Autodesk Fusion 360 part; units mm, degrees
note: some values were not read from the file. Set by a fixed rule: which face or edge a step refers to.
(part 2 of 2)
sketch "Sketch1 (3)" plane through (-90, 0, 0) normal (-1, 0, 0) x (0, -1, 0) in component "Connectors Mount"
  line L0 (67.5, -5.0963) -> (65.4615, 0)
  line L1 (65.4615, 0) -> (-61, 0)
  line L2 (-61, 0) -> (-61, -7.8)
  line L3 (-61, -7.8) -> (4, -7.8)
  line L4 (4, -7.8) -> (4, -5.8)
  line L5 (4, -5.8) -> (8.5, -5.8)
  line L6 (54, -5.8) -> (54, -7.8)
  line L7 (54, -7.8) -> (65, -7.8)
  line L8 (65, -7.8) -> (65, -15)
  line L9 (65, -15) -> (67.5, -15)
  line L10 (67.5, -15) -> (67.5, -5.0963)
  circle A0 centre (30, -3) radius 1.425
  circle A1 centre (-30, -3) radius 1.425
  line L11 (4, -7.8) -> (4, -15)
  line L12 (4, -7.8) -> (4, 0)
  line L13 (54, -7.8) -> (54, -15)
  line L14 (54, -15) -> (4, -15)
  line L15 (54, -7.8) -> (54, 0)
  circle A2 centre (30, -3) radius 1.65
  arc A3 (8.5, -5.8) -> (9, -5.3) centre (8.5, -5.3) ccw
  arc A4 (9.5, -4.8) -> (9, -5.3) centre (9.5, -5.3) ccw
  line L16 (9.5, -4.8) -> (18.5, -4.8)
  arc A5 (19, -5.3) -> (18.5, -4.8) centre (18.5, -5.3) ccw
  arc A6 (19, -5.3) -> (19.5, -5.8) centre (19.5, -5.3) ccw
  line L17 (19.5, -5.8) -> (54, -5.8)
  line L18 (4, -11.5) -> (54, -11.5)
  dimension "d86" = 3.3
  dimension "d183" = 11.5
  constraint coincident L3.end L4.start
  constraint perpendicular L3 L11
  constraint coincident L1 L12.end
  constraint perpendicular L1 L12
  constraint coincident L6.end L7.start
  constraint perpendicular L7 L13
  constraint perpendicular L6 L14
  constraint collinear L9 L14
  constraint coincident L1 L15.end
  constraint perpendicular L1 L15
  constraint concentric A0 A2
  constraint coincident L11 L18.start
  constraint coincident L13 L18.end
  constraint perpendicular L13 L18
  measures "d86" diameter of A2
  measures "d183" distance of L1 L18
extrude "Extrude1''" add sketch "Sketch1 (3)" along normal up to surface (18.55 mm away) separate body contours L1 L5 L12 L15 A3 A4 L16 A5 A6 L17 | L4 L5 L6 L11 L12 L13 L15 A3 A4 L16 A5 A6 L17 L18 makes body 3 in component "Connectors Mount"
sketch "Sketch2 (2)" plane through (-90, 0, 0) normal (1, 0, 0) x (0, 1, 0) in component "Connectors Mount"
  line L0 (-4, -11.5) -> (-4, 0)
  line L1 (-4, 0) -> (-54, 0)
  line L2 (-44.5, -11.5) -> (-44.5, -7.2)
  line L3 (-44.5, -7.2) -> (-20.2, -7.2)
  line L4 (-19.3, -5.5) -> (-9, -5.5)
  line L5 (-9, -5.5) -> (-9, -15)
  line L6 (-20.2, -7.2) -> (-20.2, -11.5)
  line L7 (-19.3, -5.5) -> (-19.3, -11.5)
  line L8 (-54, 0) -> (-54, -11.5)
  line L9 (-54, -11.5) -> (-4, -11.5)
  circle A0 centre (-30, -3) radius 1.65
  dimension "d89" = 7.2
  dimension "d92" = 5.5
  dimension "d106" = 24.3
  dimension "d107" = 35.5
  dimension "d108" = 10.3
  dimension "d184" = 9.5
  constraint perpendicular L2 L3
  constraint coincident L2.start L9
  constraint coincident L6.end L9
  constraint perpendicular L6 L9
  constraint coincident L7.end L9
  constraint perpendicular L7 L9
  measures "d89" distance of L1 L3
  measures "d92" distance of L1 L4
  measures "d106" distance of L2.end L3.end
  measures "d107" distance of L2 L5
  measures "d108" distance of L4.start L4.end
  measures "d184" distance of L2 L8
extrude "Extrude2'" cut sketch "Sketch2 (2)" against normal up to surface (18.55 mm away) contours L4 L5 L7 L9 | L2 L3 L6 L9 bodies 3 in component "Connectors Mount"
sketch "Sketch3 (3)" plane through (-108.55, 0, 0) normal (-1, 0, 0) x (0, -1, 0) in component "Connectors Mount"
  line L0 (9, -11.5) -> (9, -5.5)
  line L1 (9, -5.5) -> (19.3, -5.5)
  line L2 (19.3, -5.5) -> (19.3, -11.5)
  line L3 (20.2, -11.5) -> (20.2, -7.2)
  line L4 (20.2, -7.2) -> (44.5, -7.2)
  line L5 (44.5, -7.2) -> (44.5, -11.5)
  line L6 (54, 0) -> (4, 0)
  line L7 (4, 0) -> (4, -11.5)
  line L8 (19.3, -11.5) -> (20.2, -11.5)
  line L9 (44.5, -11.5) -> (54, -11.5)
  line L10 (54, -11.5) -> (54, 0)
  line L11 (4, -11.5) -> (9, -11.5)
  line L12 (21.7, -11.5) -> (20.2, -11.5)
  arc A0 (23.2, -8.5) -> (21.7, -10) centre (23.2, -10) ccw
  line L13 (21.7, -10) -> (21.7, -11.5)
  circle A1 centre (30, -3) radius 1.65
  line L14 (23.2, -8.5) -> (26.2, -8.5)
  line L15 (26.2, -8.5) -> (26.2, -7.2)
  dimension "d186" = 1.5
  dimension "d188" = 3
  dimension "d217" = 1.5
  dimension "d218" = 6
  constraint coincident L3.start L8.end
  constraint perpendicular L3 L12
  constraint tangent A0 L13
  constraint perpendicular L12 L13
  constraint tangent A0 L14
  constraint coincident L4 L15.end
  constraint perpendicular L4 L15
  constraint horizontal L14
  measures "d186" radius of A0
  measures "d188" distance of L3 A0.centre
  measures "d217" distance of L12 A0.centre
  measures "d218" distance of L3 L15
extrude "Extrude3''" add sketch "Sketch3 (3)" against normal blind 1.5 contours L3 L4 L12 A0 L13 L14 L15 bodies 3 in component "Connectors Mount"
sketch "Sketch4 (3)" plane through (-108.55, 0, 0) normal (-1, 0, 0) x (0, -1, 0) in component "Connectors Mount"
  line L0 (9, -11.5) -> (9, -5.5)
  line L1 (9, -5.5) -> (19.3, -5.5)
  line L2 (19.3, -5.5) -> (19.3, -11.5)
  line L3 (54, 0) -> (4, 0)
  line L4 (4, 0) -> (4, -11.5)
  circle A0 centre (14.15, -8.5) radius 3.5
  line L5 (14.15, -5.5) -> (14.15, -8.5) construction
  line L6 (17.65, -8.5) -> (17.65, -11.5201)
  line L7 (17.65, -11.5201) -> (19.3, -11.5)
  line L8 (10.65, -8.5) -> (10.65, -11.5)
  line L9 (10.65, -11.5) -> (9, -11.5)
  line L10 (19.3, -11.5) -> (21.7, -11.5)
  line L11 (54, -11.5) -> (54, 0)
  line L12 (21.7, -11.5) -> (21.7, -10)
  arc A1 (23.2, -8.5) -> (21.7, -10) centre (23.2, -10) ccw
  line L13 (23.2, -8.5) -> (26.2, -8.5)
  line L14 (26.2, -8.5) -> (26.2, -7.2)
  line L15 (26.2, -7.2) -> (44.5, -7.2)
  line L16 (44.5, -7.2) -> (44.5, -11.5)
  line L17 (44.5, -11.5) -> (54, -11.5)
  line L18 (4, -11.5) -> (9, -11.5)
  circle A2 centre (30, -3) radius 1.65
  dimension "d121" = 7
  dimension "d122" = 3
  constraint midpoint L1 L5.start
  constraint coincident A0.centre L5.end
  constraint perpendicular L1 L5
  constraint coincident A0 L6.start
  constraint perpendicular L1 L6
  constraint coincident L2.end L7.end
  constraint coincident A0 L8.start
  constraint coincident L0.start L9.end
  constraint perpendicular L0 L9
  constraint tangent A0 L8
  constraint tangent A0 L6
  measures "d121" diameter of A0
  measures "d122" distance of L5.start A0.centre
extrude "Extrude5''" cut sketch "Sketch4 (3)" against normal blind 15 contours L1 A0 picked at (14.4477, -5.2721) bodies 3 in component "Connectors Mount"
sketch "Sketch5 (3)" plane through (0, -20.2, 0) normal (0, -1, 0) x (1, 0, 0) in component "Connectors Mount"
  line L0 (-107.05, -11.5) -> (-90, -11.5)
  line L1 (-90, -11.5) -> (-90, -7.2)
  line L2 (-90, -7.2) -> (-107.05, -7.2)
  line L3 (-91, -7.2) -> (-91, -11.5)
  line L4 (-107.05, -7.2) -> (-107.05, -11.5)
  dimension "d192" = 1
  constraint coincident L2 L3.start
  constraint coincident L0 L3.end
  constraint perpendicular L0 L3
  measures "d192" distance of L1 L3
extrude "Extrude6''" add sketch "Sketch5 (3)" along normal blind 1 contours L0 L1 L2 L3 bodies 3 in component "Connectors Mount"
fillet "Fillet8'" radius 1 8 edges at (-99.275, -54, 0) (-99.275, -4, 0) (-90, -4, -5.75) (-90, -29, 0) (-90, -54, -5.75) (-108.55, -54, -5.75) (-108.55, -29, 0) (-108.55, -4, -5.75) on bodies 3 in component "Connectors Mount"
sketch "Sketch2 (3)" plane through (0, 0, -7.8) normal (0, 0, -1) x (1, 0, 0) in component "Bottom"
  circle A0 centre (60, 60) radius 1.65
  circle A1 centre (60, -60) radius 1.65
  circle A2 centre (-60, 60) radius 1.65
  circle A3 centre (-60, -60) radius 1.65
  arc A4 (-73.75, 56) -> (-71.75, 54) centre (-71.75, 56) ccw
  line L0 (-71.75, 54) -> (71.75, 54)
  arc A5 (71.75, 54) -> (73.75, 56) centre (71.75, 56) ccw
  line L1 (73.75, 56) -> (73.75, 61)
  arc A6 (75.75, 63) -> (73.75, 61) centre (75.75, 61) ccw
  line L2 (75.75, 63) -> (86, 63)
  arc A7 (88, 61) -> (86, 63) centre (86, 61) ccw
  line L3 (88, 61) -> (88, -61)
  arc A8 (86, -63) -> (88, -61) centre (86, -61) ccw
  line L4 (86, -63) -> (75.75, -63)
  arc A9 (73.75, -61) -> (75.75, -63) centre (75.75, -61) ccw
  line L5 (73.75, -61) -> (73.75, -56)
  arc A10 (73.75, -56) -> (71.75, -54) centre (71.75, -56) ccw
  line L6 (71.75, -54) -> (-71.75, -54)
  arc A11 (-71.75, -54) -> (-73.75, -56) centre (-71.75, -56) ccw
  line L7 (-73.75, -56) -> (-73.75, -61)
  arc A12 (-75.75, -63) -> (-73.75, -61) centre (-75.75, -61) ccw
  line L8 (-75.75, -63) -> (-86, -63)
  arc A13 (-88, -61) -> (-86, -63) centre (-86, -61) ccw
  line L9 (-88, -61) -> (-88, 4)
  line L10 (-88, 4) -> (-90, 4)
  line L11 (-90, 4) -> (-90, -61)
  arc A14 (-90, -61) -> (-86, -65) centre (-86, -61) ccw
  line L12 (-86, -65) -> (86, -65)
  arc A15 (86, -65) -> (90, -61) centre (86, -61) ccw
  line L13 (90, -61) -> (90, 65)
  line L14 (90, 65) -> (-90, 65)
  line L15 (-90, 65) -> (-90, 54)
  line L16 (-90, 54) -> (-88, 54)
  line L17 (-88, 54) -> (-88, 61)
  arc A16 (-86, 63) -> (-88, 61) centre (-86, 61) ccw
  line L18 (-86, 63) -> (-75.75, 63)
  arc A17 (-73.75, 61) -> (-75.75, 63) centre (-75.75, 61) ccw
  line L19 (-73.75, 61) -> (-73.75, 56)
  circle A18 centre (78.5, 57.5) radius 1.65 construction
  circle A19 centre (78.5, 57.5) radius 1.65 construction
  circle A20 centre (-78.5, 57.5) radius 1.65 construction
  circle A21 centre (-78.5, 57.5) radius 1.65 construction
  circle A22 centre (-78.5, -57.5) radius 1.65 construction
  circle A23 centre (-78.5, -57.5) radius 1.65 construction
  circle A24 centre (78.5, -57.5) radius 1.65 construction
  circle A25 centre (78.5, -57.5) radius 1.65 construction
  circle A26 centre (-78.5, 57.5) radius 3.25
  circle A27 centre (78.5, 57.5) radius 3.25
  circle A28 centre (78.5, -57.5) radius 3.25
  circle A29 centre (-78.5, -57.5) radius 3.25
  line L20 (-81.75, 6) -> (-81.75, -51.2752)
  line L21 (-81.75, -51.2752) -> (81.75, -51.2752)
  line L22 (81.75, -51.2752) -> (81.75, 52)
  line L23 (81.75, 52) -> (-90, 52)
  line L24 (-90, 52) -> (-90, 54)
  line L25 (83.75, 53) -> (83.75, -53) construction
  line L26 (-83.75, -53) -> (-83.75, 8.5) construction
  line L27 (-81.75, 6) -> (-90, 6)
  line L28 (-90, 6) -> (-90, 4)
  dimension "d133" = 6.5
  dimension "d134" = 2
  dimension "d135" = 2
  dimension "d136" = 2.7248
  dimension "d137" = 2
  dimension "d146" = 2
  constraint concentric A20 A26
  constraint concentric A18 A27
  constraint concentric A24 A28
  constraint concentric A22 A29
  constraint equal A28 A29
  constraint equal A27 A28
  constraint equal A26 A27
  constraint perpendicular L10 L20
  constraint perpendicular L9 L21
  constraint perpendicular L6 L22
  constraint perpendicular L9 L23
  constraint coincident L15.end L16.start
  constraint collinear L15 L24
  constraint perpendicular L20 L27
  constraint coincident L10.end L11.start
  constraint collinear L11 L28
  measures "d133" diameter of A26
  measures "d134" distance of L0 L23
  measures "d135" distance of L22 L25
  measures "d136" distance of L6 L21
  measures "d137" distance of L20 L26
  measures "d146" distance of L27.end L10.end
extrude "Extrude2''" add sketch "Sketch2 (3)" along normal blind 9.5 separate body makes body 4 in component "Bottom"
sketch "Sketch3 (4)" plane through (0, 0, -17.3) normal (0, 0, -1) x (1, 0, 0) in component "Bottom"
  circle A0 centre (-60, -60) radius 1.65
  circle A1 centre (60, 60) radius 1.65
  circle A2 centre (60, -60) radius 1.65
  circle A3 centre (78.5, -57.5) radius 3.25
  circle A4 centre (-78.5, -57.5) radius 3.25
  circle A5 centre (-78.5, 57.5) radius 3.25
  circle A6 centre (78.5, 57.5) radius 3.25
  circle A7 centre (-60, 60) radius 1.65
  line L0 (-90, 4) -> (-90, -61)
  arc A8 (-90, -61) -> (-86, -65) centre (-86, -61) ccw
  line L1 (-86, -65) -> (86, -65)
  arc A9 (86, -65) -> (90, -61) centre (86, -61) ccw
  line L2 (90, -61) -> (90, 65)
  line L3 (90, 65) -> (-90, 65)
  line L4 (-90, 65) -> (-90, 54)
  line L5 (-90, 54) -> (-90, 52)
  line L6 (-90, 52) -> (81.75, 52)
  line L7 (81.75, 52) -> (81.75, -51.2752)
  line L8 (81.75, -51.2752) -> (-81.75, -51.2752)
  line L9 (-81.75, -51.2752) -> (-81.75, 6)
  line L10 (-90, 4) -> (-90, 52)
  line L11 (-81.75, 6) -> (-90, 6)
  line L12 (-90, 6) -> (-90, 4)
  constraint coincident L0.start L10.start
  constraint coincident L5.end L6.start
extrude "Extrude3'''" add sketch "Sketch3 (4)" along normal blind 3 contours A3 | A4 | A5 | A6 | L0 A8 L1 A9 L2 L3 L4 L5 L6 L7 L8 L9 L10 L11 L12 | L6 L7 L8 L9 L10 L11 bodies 4 in component "Bottom"
sketch "Sketch4 (4)" plane through (0, 0, -20.3) normal (0, 0, -1) x (1, 0, 0) in component "Bottom"
  circle A0 centre (60, 60) radius 1.65
  circle A1 centre (-60, 60) radius 1.65
  circle A2 centre (-60, -60) radius 1.65
  circle A3 centre (60, -60) radius 1.65
  arc A4 (-90, -61) -> (-86, -65) centre (-86, -61) ccw
  line L0 (-86, -65) -> (86, -65)
  arc A5 (86, -65) -> (90, -61) centre (86, -61) ccw
  line L1 (90, -61) -> (90, 65)
  line L2 (90, 65) -> (-90, 65)
  line L3 (-90, 65) -> (-90, 54)
  line L4 (-90, 54) -> (-90, 52)
  line L5 (-90, 4) -> (-90, -61)
  line L6 (-108.75, 31.65) -> (-108.75, 28.35) construction
  line L7 (-108.75, 54) -> (-108.75, 4) construction
  line L8 (-108.75, 4) -> (-108.75, 54) construction
  line L9 (-108.75, 54) -> (-108.75, 4)
  line L10 (-108.75, 4) -> (-90, 4)
  line L11 (-90.6, 4) -> (-108.75, 4) construction
  circle A6 centre (-99.375, 49) radius 1.65
  circle A7 centre (-99.375, 9) radius 1.65
  line L12 (-108.75, 29) -> (-95, 29) construction
  line L13 (-99.375, 4) -> (-99.375, 29.3924) construction
  line L14 (-90, 6) -> (-90, 4)
  line L15 (-108.75, 54) -> (-90, 54)
  line L16 (-90, 52) -> (-90, 6)
  dimension "d142" = 40
  dimension "d143" = 3.3
  constraint perpendicular L2 L9
  constraint collinear L10 L11
  constraint collinear L8 L9
  constraint midpoint L9 L12.start
  constraint perpendicular L7 L12
  constraint midpoint L10 L13.start
  constraint coincident A7.centre L13
  constraint symmetric A6 A7 L12
  constraint coincident L7.start L8.end
  constraint coincident L3.end L4.start
  constraint vertical L13
  constraint coincident L5.start L10.end
  measures "d142" distance of A6.centre A7.centre
  measures "d143" diameter of A7
extrude "Extrude4''" add sketch "Sketch4 (4)" against normal up to surface (3 mm away) contours L4 L9 L10 L14 L15 L16 bodies 4 in component "Bottom"
fillet "Fillet1'" radius 4 1 edges at (90, -65, -14.05) on bodies 4 in component "Bottom"
sketch "Sketch5 (4)" plane through (0, 0, -17.3) normal (0, 0, 1) x (-1, 0, 0) in component "Bottom"
  line L0 (108.75, 4) -> (108.75, 54)
  line L1 (90, 54) -> (90, 52)
  line L2 (90, 52) -> (-81.75, 52)
  line L3 (-81.75, 52) -> (-81.75, -51.2752)
  line L4 (-81.75, -51.2752) -> (81.75, -51.2752)
  line L5 (81.75, -51.2752) -> (81.75, 6)
  line L6 (81.75, 6) -> (90, 6)
  line L7 (90, 6) -> (90, 4)
  line L8 (90, 4) -> (108.75, 4)
  circle A0 centre (99.375, 49) radius 1.65
  circle A1 centre (99.375, 9) radius 1.65
  circle A2 centre (19, -24.5) radius 1.375
  circle A3 centre (-39, -24.5) radius 1.375
  circle A4 centre (-39, 24.5) radius 1.375
  circle A5 centre (19, 24.5) radius 1.375
  circle A6 centre (19, 24.5) radius 2.5
  circle A7 centre (-39, 24.5) radius 2.5
  circle A8 centre (-39, -24.5) radius 2.5
  circle A9 centre (19, -24.5) radius 2.5
  line L9 (108.75, 54) -> (90, 54)
  dimension "d151" = 19
  dimension "d152" = 39
  dimension "d154" = 24.5
  dimension "d155" = 24.5
  dimension "d156" = 2.75
  dimension "d170" = 5
  constraint horizontal A2.centre A3.centre
  constraint equal A4 A5
  constraint equal A3 A4
  constraint equal A2 A3
  constraint vertical A2.centre A5.centre
  constraint vertical A3.centre A4.centre
  constraint horizontal A4.centre A5.centre
  constraint concentric A5 A6
  constraint concentric A4 A7
  constraint concentric A3 A8
  constraint concentric A2 A9
  constraint equal A8 A9
  constraint equal A7 A8
  constraint equal A6 A7
  measures "d151" horizontal distance of origin A2.centre
  measures "d152" horizontal distance of origin A3.centre
  measures "d154" vertical distance of origin A3.centre
  measures "d155" vertical distance of origin A4.centre
  measures "d156" diameter of A5
  measures "d170" diameter of A6
extrude "Extrude5'''" cut sketch "Sketch5 (4)" against normal up to surface (3 mm away) contours A2 | A3 | A4 | A5 bodies 4 in component "Bottom"
extrude "Extrude8'" add sketch "Sketch5 (4)" along normal up to surface (3.5 mm away) contours A6 | A7 | A8 | A9 bodies 4 in component "Bottom"
sketch "Sketch8 (2)" plane through (0, 0, -20.3) normal (0, 0, -1) x (1, 0, 0) in component "Bottom"
  circle A0 centre (-19, 24.5) radius 1.375
  circle A1 centre (39, 24.5) radius 1.375
  circle A2 centre (-19, -24.5) radius 1.375
  circle A3 centre (39, -24.5) radius 1.375
  arc A4 (90, 61) -> (86, 65) centre (86, 61) ccw
  line L0 (86, 65) -> (-90, 65)
  line L1 (-90, 65) -> (-90, 54)
  line L2 (-90, 54) -> (-108.75, 54)
  line L3 (-108.75, 54) -> (-108.75, 4)
  line L4 (-108.75, 4) -> (-90, 4)
  line L5 (-90, 4) -> (-90, -61)
  arc A5 (-90, -61) -> (-86, -65) centre (-86, -61) ccw
  line L6 (-86, -65) -> (86, -65)
  arc A6 (86, -65) -> (90, -61) centre (86, -61) ccw
  line L7 (90, -61) -> (90, 61)
  circle A7 centre (-60, -60) radius 1.65
  circle A8 centre (60, 60) radius 1.65
  circle A9 centre (-60, 60) radius 1.65
  circle A10 centre (60, -60) radius 1.65
  circle A11 centre (-99.375, 49) radius 1.65
  circle A12 centre (-99.375, 9) radius 1.65
  circle A13 centre (39, 24.5) radius 2.5
  circle A14 centre (-19, 24.5) radius 2.5
  circle A15 centre (-19, -24.5) radius 2.5
  circle A16 centre (39, -24.5) radius 2.5
  dimension "d213" = 5
  constraint concentric A1 A13
  constraint concentric A0 A14
  constraint concentric A2 A15
  constraint concentric A3 A16
  constraint equal A13 A14
  constraint equal A14 A15
  constraint equal A15 A16
  measures "d213" diameter of A13
extrude "Extrude10'" cut sketch "Sketch8 (2)" against normal up to surface (2.5 mm away) contours A13 | A14 | A15 | A16 bodies 4 in component "Bottom"
sketch "Sketch6 (2)" plane through (0, 0, -17.3) normal (0, 0, 1) x (-1, 0, 0) in component "Bottom"
  line L0 (108.75, 4) -> (108.75, 54)
  line L1 (90, 54) -> (90, 52)
  line L2 (90, 52) -> (-81.75, 52)
  line L3 (-81.75, 52) -> (-81.75, -51.2752)
  line L4 (-81.75, -51.2752) -> (81.75, -51.2752)
  line L5 (81.75, -51.2752) -> (81.75, 6)
  line L6 (81.75, 6) -> (90, 6)
  line L7 (90, 6) -> (90, 4)
  line L8 (90, 4) -> (108.75, 4)
  circle A0 centre (99.375, 49) radius 1.65
  circle A1 centre (99.375, 9) radius 1.65
  line L9 (25, -20) -> (-25, -20) construction
  line L10 (-25, -20) -> (-25, 20) construction
  line L11 (-25, 20) -> (25, 20) construction
  line L12 (25, 20) -> (25, -20) construction
  line L13 (0, 0) -> (-48.8562, 0) construction
  circle A2 centre (-25, -20) radius 4
  circle A3 centre (-25, 20) radius 4
  line L14 (0, 0) -> (0, -41.4646) construction
  circle A4 centre (-19, -24.5) radius 2.75 construction
  circle A5 centre (25, -20) radius 4
  circle A6 centre (25, 20) radius 4
  circle A7 centre (-25, -20) radius 1.65
  circle A8 centre (-25, 20) radius 1.65
  circle A9 centre (25, 20) radius 1.65
  circle A10 centre (25, -20) radius 1.65
  line L15 (-26.5588, -17.3) -> (-28.1177, -20)
  line L16 (-28.1177, -20) -> (-26.5588, -22.7)
  line L17 (-26.5588, -22.7) -> (-23.4412, -22.7)
  line L18 (-23.4412, -22.7) -> (-21.8823, -20)
  line L19 (-21.8823, -20) -> (-23.4412, -17.3)
  line L20 (-23.4412, -17.3) -> (-26.5588, -17.3)
  line L21 (23.4412, -17.3) -> (21.8823, -20)
  line L22 (21.8823, -20) -> (23.4412, -22.7)
  line L23 (23.4412, -22.7) -> (26.5588, -22.7)
  line L24 (26.5588, -22.7) -> (28.1177, -20)
  line L25 (28.1177, -20) -> (26.5588, -17.3)
  line L26 (26.5588, -17.3) -> (23.4412, -17.3)
  line L27 (23.4412, 22.7) -> (21.8823, 20)
  line L28 (21.8823, 20) -> (23.4412, 17.3)
  line L29 (23.4412, 17.3) -> (26.5588, 17.3)
  line L30 (26.5588, 17.3) -> (28.1177, 20)
  line L31 (28.1177, 20) -> (26.5588, 22.7)
  line L32 (26.5588, 22.7) -> (23.4412, 22.7)
  line L33 (-26.5588, 22.7) -> (-28.1177, 20)
  line L34 (-28.1177, 20) -> (-26.5588, 17.3)
  line L35 (-26.5588, 17.3) -> (-23.4412, 17.3)
  line L36 (-23.4412, 17.3) -> (-21.8823, 20)
  line L37 (-21.8823, 20) -> (-23.4412, 22.7)
  line L38 (-23.4412, 22.7) -> (-26.5588, 22.7)
  circle A11 centre (-39, -24.5) radius 2.5
  circle A12 centre (19, -24.5) radius 2.5
  circle A13 centre (-39, 24.5) radius 2.5
  circle A14 centre (19, 24.5) radius 2.5
  line L39 (108.75, 54) -> (90, 54)
  point P0 (-25, -20)
  point P1 (25, -20)
  point P2 (25, 20)
  point P3 (-25, 20)
  dimension "d159" = 50
  dimension "d160" = 8
  dimension "d162" = 40
  dimension "d163" = 5.5
  dimension "d164" = 3.3
  dimension "d167" = 2.7
  constraint horizontal L9
  constraint vertical L10
  constraint horizontal L11
  constraint vertical L12
  constraint coincident L13.start L14.start
  constraint horizontal L13
  constraint symmetric L9 L11 L13
  constraint coincident P0 L9.end
  constraint coincident P3 L10.end
  constraint perpendicular L13 L14
  constraint symmetric L10 L12 L14
  constraint coincident P1 L9.start
  constraint coincident P2 L11.end
  constraint concentric A2 A7
  constraint equal A2 A3
  constraint equal A3 A6
  constraint equal A5 A6
  constraint concentric A3 A8
  constraint concentric A6 A9
  constraint concentric A5 A10
  constraint equal A7 A10
  constraint equal A9 A10
  constraint equal A8 A9
  constraint horizontal L20
  constraint equal L32 L38
  constraint equal L26 L32
  constraint equal L20 L26
  constraint horizontal L26
  constraint horizontal L32
  constraint horizontal L38
  measures "d159" distance of P1 P0
  measures "d160" diameter of A2
  measures "d162" distance of P0 P3
  measures "d163" diameter of A4
  measures "d164" diameter of A7
  measures "d167" distance of P0 L20
extrude "Extrude6'''" cut sketch "Sketch6 (2)" against normal up to surface (3 mm away) contours A7 | A8 | A9 | A10 bodies 4 in component "Bottom"
extrude "Extrude7'" add sketch "Sketch6 (2)" along normal blind 3 contours A2 | A3 | A5 | A6 bodies 4 in component "Bottom"
sketch "Sketch7 (2)" plane through (0, 0, -17.3) normal (0, 0, 1) x (-1, 0, 0) in component "Bottom"
  circle A0 centre (25, 20) radius 4
  circle A1 centre (-25, 20) radius 4
  circle A2 centre (-39, -24.5) radius 2.5
  circle A3 centre (19, -24.5) radius 2.5
  circle A4 centre (-39, 24.5) radius 2.5
  circle A5 centre (19, 24.5) radius 2.5
  line L0 (108.75, 4) -> (108.75, 54)
  line L1 (90, 54) -> (90, 52)
  line L2 (90, 52) -> (-81.75, 52)
  line L3 (-81.75, 52) -> (-81.75, -51.2752)
  line L4 (-81.75, -51.2752) -> (81.75, -51.2752)
  line L5 (81.75, -51.2752) -> (81.75, 6)
  line L6 (81.75, 6) -> (90, 6)
  line L7 (90, 6) -> (90, 4)
  line L8 (90, 4) -> (108.75, 4)
  circle A6 centre (99.375, 49) radius 1.65
  circle A7 centre (99.375, 9) radius 1.65
  circle A8 centre (-25, -20) radius 4
  circle A9 centre (25, -20) radius 4
  line L9 (-21, -51.2752) -> (-21, 52)
  line L10 (-29, 52) -> (-29, -51.2752)
  line L11 (29, -51.2752) -> (29, 52)
  line L12 (21, 52) -> (21, -51.2752)
  line L13 (108.75, 54) -> (90, 54)
  constraint coincident L4 L9.start
  constraint coincident L2 L9.end
  constraint coincident L2 L10.start
  constraint coincident L4 L10.end
  constraint perpendicular L4 L10
  constraint coincident L4 L11.start
  constraint coincident L2 L11.end
  constraint perpendicular L2 L11
  constraint coincident L2 L12.start
  constraint coincident L4 L12.end
  constraint perpendicular L4 L12
  constraint perpendicular L4 L9
  constraint tangent A8 L9
  constraint tangent A8 L10
  constraint tangent A9 L12
  constraint tangent A9 L11
extrude "Extrude9'" add sketch "Sketch7 (2)" along normal blind 2 contours A0 A9 L11 L12 | A0 A5 L2 L11 L12 | A3 L4 A9 L11 L12 | A5 L12 | A3 L12 | A1 L2 L9 L10 | L4 A8 L9 L10 | A1 A8 L9 L10 picked at (21.2565, 24.2879) picked at (21.2565, -24.7121) bodies 4 in component "Bottom"
fillet "Fillet3'" radius 2 4 edges at (-81.75, 51.2752, -12.55) (-81.75, -6, -12.55) (81.75, 51.2752, -12.55) (81.75, -52, -12.55) on bodies 4 in component "Bottom"
fillet "Fillet4'" radius 1 9 edges at (-29, -0.3624, -17.3) (-59.5, -52, -17.3) (-54.375, 51.2752, -17.3) (-81.1642, 50.6894, -17.3) (-81.75, 22.6376, -17.3) (-82.3358, -5.4142, -17.3) (-86.875, -6, -17.3) (-16.6692, 23.596, -17.3) (-16.6692, -25.404, -17.3) 2 faces at (8.4203, -8.0527, -17.3) (68.2508, -8.0467, -17.3) on bodies 4 in component "Bottom"
fillet "Fillet5" radius 1 8 edges at (25, 16, -15.3) (25, -24, -15.3) (-25, -24, -15.3) (-25, 16, -15.3) (25, 24, -15.3) (-25, 24, -15.3) (-25, -16, -15.3) (25, -16, -15.3) on bodies 4 in component "Bottom"
sketch "Sketch1 (4)" plane through (-108.75, 0, 0) normal (-1, 0, 0) x (0, -1, 0) in component "Connectors Mount Bottom"
  line L0 (54, -17.3) -> (4, -17.3)
  line L1 (4, -17.3) -> (4, -20.3)
  line L2 (4, -20.3) -> (54, -20.3)
  line L3 (54, -20.3) -> (54, -17.3)
  arc A0 (15.9528, -5.5) -> (12.3472, -5.5) centre (14.15, -8.5) ccw
  arc A1 (23.2, -8.5) -> (21.7, -10) centre (23.2, -10) ccw
  line L4 (21.7, -10) -> (21.7, -11.5)
  line L5 (54, -17.3) -> (54, -11.5)
  circle A2 centre (14.15, -8.5) radius 3.5
  line L6 (21.7, -11.5) -> (15.9528, -11.5)
  line L7 (12.3472, -11.5) -> (4, -11.5)
  line L8 (4, -11.5) -> (4, -17.3)
  line L9 (23.2, -8.5) -> (26.2, -8.5)
  line L10 (26.2, -8.5) -> (26.2, -7.2)
  line L11 (26.2, -7.2) -> (44.5, -7.2)
  line L12 (44.5, -7.2) -> (44.5, -11.5)
  line L13 (21.7, -13) -> (21.7, -11.5)
  arc A3 (21.7, -13) -> (23.2, -14.5) centre (23.2, -13) ccw
  line L14 (23.2, -14.5) -> (26.2, -14.5)
  line L15 (26.2, -14.5) -> (26.2, -15.8)
  line L16 (26.2, -15.8) -> (44.5, -15.8)
  line L17 (44.5, -15.8) -> (44.5, -11.5)
  line L18 (44.5, -11.5) -> (54, -11.5)
  constraint coincident L0.start L3.end
  constraint perpendicular L0 L5
  constraint concentric A0 A2
  constraint equal A0 A2
  constraint coincident L4.end L6.start
  constraint coincident A2 L6.end
  constraint perpendicular L4 L6
  constraint coincident A2 L7.start
  constraint horizontal L7
  constraint coincident L0.end L1.start
  constraint collinear L6 L7
  constraint perpendicular L7 L8
  constraint symmetric A1.start L6 A3.end
  constraint symmetric A1.end L6 L13.start
  constraint symmetric A1 L6 A3
  constraint symmetric L4.end L6 L13.end
  constraint symmetric L6 A1.start A3.end
  constraint symmetric L6 L9.end L14.end
  constraint symmetric L6 L10.end L15.end
  constraint symmetric L6 L11.end L16.end
  constraint symmetric L6 L12.end L17.end
  constraint coincident L12.end L17.end
  constraint perpendicular L5 L18
extrude "Extrude1'''" add sketch "Sketch1 (4)" against normal up to surface (18.75 mm away) separate body contours L0 L5 A2 L6 L7 L8 L13 A3 L14 L15 L16 L17 L18 makes body 5 in component "Connectors Mount Bottom"
sketch "Sketch2 (4)" plane through (0, 0, -17.3) normal (0, 0, -1) x (1, 0, 0) in component "Connectors Mount Bottom"
  line L0 (-90, 4) -> (-90, 54)
  line L1 (-90, 54) -> (-108.75, 54)
  line L2 (-108.75, 54) -> (-108.75, 4)
  line L3 (-108.75, 4) -> (-90, 4)
  circle A0 centre (-99.375, 9) radius 1.65 construction
  circle A1 centre (-99.375, 9) radius 1.65 construction
  circle A2 centre (-99.375, 49) radius 1.65 construction
  circle A3 centre (-99.375, 49) radius 1.65 construction
  circle A4 centre (-99.375, 9) radius 1.425
  circle A5 centre (-99.375, 49) radius 1.425
  dimension "d198" = 2.85
  constraint concentric A0 A4
  constraint concentric A2 A5
  constraint equal A4 A5
  measures "d198" diameter of A4
extrude "Extrude2'''" cut sketch "Sketch2 (4)" against normal up to surface (5.3 mm away) contours A4 | A5 bodies 5 in component "Connectors Mount Bottom"
sketch "Sketch4 (5)" plane through (-90, 0, 0) normal (1, 0, 0) x (0, 1, 0) in component "Connectors Mount Bottom"
  line L0 (-15.9528, -11.5) -> (-21.7, -11.5)
  line L1 (-21.7, -11.5) -> (-21.7, -13)
  arc A0 (-23.2, -14.5) -> (-21.7, -13) centre (-23.2, -13) ccw
  line L2 (-23.2, -14.5) -> (-26.2, -14.5)
  line L3 (-26.2, -14.5) -> (-26.2, -15.8)
  line L4 (-26.2, -15.8) -> (-44.5, -15.8)
  line L5 (-44.5, -15.8) -> (-44.5, -11.5)
  line L6 (-44.5, -11.5) -> (-54, -11.5)
  line L7 (-54, -11.5) -> (-54, -17.3)
  line L8 (-54, -17.3) -> (-4, -17.3)
  line L9 (-4, -17.3) -> (-4, -11.5)
  line L10 (-4, -11.5) -> (-12.3472, -11.5)
  arc A1 (-15.9528, -11.5) -> (-12.3472, -11.5) centre (-14.15, -8.5) ccw
  line L11 (-20.2, -11.5) -> (-20.2, -7.2)
  line L12 (-20.2, -7.2) -> (-20.2, -11.5)
  line L13 (-20.2, -11.5) -> (-20.2, -15.8)
  line L14 (-20.2, -15.8) -> (-26.2, -15.8)
  constraint coincident L11.start L12.end
  constraint perpendicular L0 L13
  constraint coincident L3.end L4.start
  constraint perpendicular L13 L14
extrude "Extrude4'''" cut sketch "Sketch4 (5)" against normal up to surface (17.05 mm away) contours L0 L1 A0 L2 L3 L13 L14 bodies 5 in component "Connectors Mount Bottom"
fillet "Fillet2'" radius 1 4 edges at (-108.75, -4, -14.4) (-90, -4, -14.4) (-108.75, -54, -14.4) (-90, -54, -14.4) on bodies 5 in component "Connectors Mount Bottom"
fillet "Fillet6" radius 1 4 edges at (-108.75, -54, -18.8) (-90, -54, -18.8) (-108.75, -4, -18.8) (-90, -4, -18.8) on bodies 4 in component "Bottom"
chamfer "Chamfer2" distance 1.5 distance2 1.5 4 edges at (-61.5383, -60.5967, -20.3) (-61.5383, 59.4033, -20.3) (58.4617, 59.4033, -20.3) (58.4617, -60.5967, -20.3) measured on face at (73.7771, 7.8656, -20.3) measured on face at (73.7771, 7.8656, -20.3) measured on face at (73.7771, 7.8656, -20.3) measured on face at (73.7771, 7.8656, -20.3) on bodies 4 in component "Bottom"
component "Main Body" placed x (1, 0, 0) y (0, 1, 0) z (0, 0, 1) at (0, 0, 0)
component "Top Cover" placed x (1, 0, 0) y (0, 1, 0) z (0, 0, 1) at (0, 0, 0)
component "Connectors Mount" placed x (1, 0, 0) y (0, 1, 0) z (0, 0, 1) at (0, 0, 0)
component "Bottom" placed x (1, 0, 0) y (0, 1, 0) z (0, 0, 1) at (0, 0, 0)
component "Connectors Mount Bottom" placed x (1, 0, 0) y (0, 1, 0) z (0, 0, 1) at (0, 0, 0)

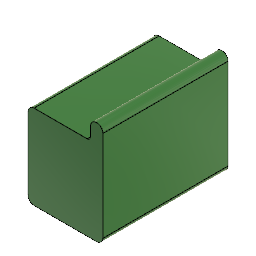
design "Spacer"
Autodesk Fusion 360 part; units mm, degrees
sketch "Sketch1" plane through (0, 0, 0) normal (0, 1, 0) x (1, 0, 0)
  line L0 (0, 0) -> (0, -3)
  line L1 (0, -3) -> (2, -3)
  line L2 (2, -3) -> (2, 13.5)
  line L3 (2, 13.5) -> (-10, 13.5)
  line L4 (-10, 13.5) -> (-10, 0)
  line L5 (-10, 0) -> (0, 0)
  dimension "d1" = 3
  dimension "d2" = 10
  dimension "d4" = 13.5
  dimension "d5" = 2
  constraint coincident L0.start L5.end
  constraint vertical L0
  constraint perpendicular L0 L1
  constraint perpendicular L1 L2
  constraint perpendicular L2 L3
  constraint perpendicular L3 L4
  constraint perpendicular L0 L5
  measures "d1" distance of L0.start L0.end
  measures "d2" distance of L4.end L0.start
  measures "d4" distance of L3.end L4.end
  measures "d5" distance of L0.end L1.end
extrude "Extrude1" add sketch "Sketch1" along normal mid plane 20
fillet "Fillet1" radius 1 5 edges at (2, 0, -13.5) (-10, 0, -13.5) (-10, 0, 0) (2, 0, 3) (0, 0, 3)
fillet "Fillet2" radius 0.5 1 edges at (0, 0, 0)
